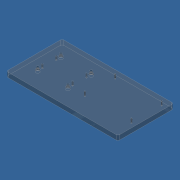
# Autodesk Inventor part: Paddle_Base
Saved by Autodesk Inventor 2011 SP1 (Build 150282100, 282)
## iProperties
Created: 2011-08-29
Part Number: Paddle_Base
Document SubType Name: Modeling
Designer: wespep
Density: 1 g/cm^3
Author: wespep
Autodesk Inventor part; units mm, degrees
ref_plane "YZ Plane" through (0, 0, 0) normal (1, 0, 0) x (0, 1, 0)
ref_plane "XZ Plane" through (0, 0, 0) normal (0, 1, 0) x (-1, 0, 0)
ref_plane "XY Plane" through (0, 0, 0) normal (0, 0, 1) x (1, 0, 0)
sketch "Skizze1" plane through (0, 0, 0) normal (0, 0, 1) x (1, 0, 0)
  line L0 (0, 0) -> (95, 0)
  line L1 (95, 0) -> (95, 120)
  line L2 (95, 120) -> (0, 120)
  line L3 (0, 120) -> (0, 0)
  circle A0 centre (38.1, 37.9782) radius 2.905
  circle A1 centre (90, 42.5) radius 1.5
  circle A2 centre (24.7598, 24.638) radius 2.905
  circle A3 centre (38.1, 11.2978) radius 2.905
  circle A4 centre (51.4402, 24.638) radius 2.905
  circle A5 centre (90, 92.5) radius 1.5
  circle A6 centre (25, 42.5) radius 1.5
  circle A7 centre (25, 92.5) radius 1.5
  line L4 (0, 120) -> (240, 120)
  line L5 (240, 120) -> (240, 0)
  line L6 (240, 0) -> (0, 0)
  line L7 (0, 0) -> (0, 120)
  circle A8 centre (222, 112) radius 1.5
  circle A9 centre (122, 112) radius 1.5
  circle A10 centre (222, 47) radius 1.5
  circle A11 centre (122, 47) radius 1.5
  point P0 (38.1, 24.638)
  dimension "d0" = 120
  dimension "d1" = 95
  dimension "d5" = 5
  dimension "d6" = 3
  dimension "d12" = 360
  dimension "d16" = 50
  dimension "d19" = 65
  dimension "d69" = 42.5
  dimension "d99" = 240
  dimension "d100" = 120
  dimension "d103" = 8
  dimension "d104" = 18
  dimension "d105" = 3
  dimension "d108" = 100
  dimension "d111" = 65
  dimension "d114" = 47
  constraints: 16 end point, 12 centre point, 4 horizontal, 4 parallel, 2 perpendicular, 2 vertical, 21 other
  measures "d0" distance of L2.end L0.start
  measures "d1" distance of L0.start L0.end
  measures "d5" distance from line of L1 A1.centre
  measures "d6" diameter of A1
  measures "d16" distance of A1.centre A5.centre
  measures "d19" distance of A1.centre A6.centre
  measures "d69" distance from line of A1.centre L0
  measures "d99" distance of L2.end L4.end
  measures "d100" distance of L4.end L5.end
  measures "d103" distance from line of L4 A8.centre
  measures "d104" distance from line of L5 A8.centre
  measures "d105" diameter of A8
  measures "d108" distance of A8.centre A9.centre
  measures "d111" distance of A8.centre A10.centre
  measures "d114" distance from line of L6 A10.centre
extrude "Extrusion2" add sketch "Skizze1" against normal blind 10 contours L3 L2 L1 L0 | L1 L4 L5 L6 | A0 | A2 | A3 | A4 | A8 | A9 | A10 | A11
hole "Bohrung8" at (122, 112, 0) at (222, 112, 0) at (222, 47, 0) at (122, 47, 0) direction (0, 0, -1) diameter 2.459 depth 9 tip angle 118 thread size "M3x0.5" class "6H" standard "ISO Metric profile"
sketch "Skizze11" plane through (0, 0, -10) normal (0, 0, -1) x (-1, 0, 0)
  circle A0 centre (-25, 92.5) radius 1.5 projected
  circle A1 centre (-25, 42.5) radius 1.5 projected
  circle A2 centre (-90, 92.5) radius 1.5 projected
  circle A3 centre (-90, 42.5) radius 1.5 projected
hole "Bohrung11" at (25, 42.5, -10) at (90, 42.5, -10) at (90, 92.5, -10) at (25, 92.5, -10) direction (0, 0, 1) diameter 4.3 depth 13 tip angle 118 counterbore diameter 7.5 counterbore depth 4.5
sketch "Skizze12" plane through (0, 0, 0) normal (0, 0, 1) x (1, 0, 0)
  circle A0 centre (25, 92.5) radius 2.15 projected
  circle A1 centre (25, 42.5) radius 2.15 projected
  line L0 (240, 120) -> (0, 120) projected
  line L1 (25, 92.5) -> (25, 42.5)
  circle A2 centre (25, 82.5) radius 1.5
  circle A3 centre (25, 52.5) radius 1.5
  circle A4 centre (90, 82.5) radius 1.5
  circle A5 centre (90, 52.5) radius 1.5
  dimension "d163" = 3
  dimension "d164" = 10
  dimension "d167" = 30
  dimension "d170" = 65
  constraints: 4 centre point, 2 end point, 1 horizontal, 1 perpendicular, 1 point on line, 1 vertical, 6 other
  measures "d163" diameter of A2
  measures "d164" distance of A2.centre L1.start
  measures "d167" distance of A2.centre A3.centre
  measures "d170" distance of A2.centre A4.centre
hole "Bohrung12" at (25, 82.5, 0) at (25, 52.5, 0) at (90, 52.5, 0) at (90, 82.5, 0) direction (0, 0, -1) diameter 3 depth 8 tip angle 118
fillet "Rundung1" radius 4 4 edges at (240, 0, -5) (0, 0, -5) (0, 120, -5) (240, 120, -5)
equation "\"d100\" = d0"
